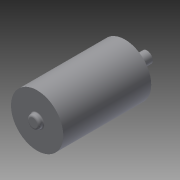
# Autodesk Inventor part: motor
Saved by Autodesk Inventor 2014 SP1 (Build 180222100, 222)
## iProperties
Created: 2014-09-21
Part Number: motor
Material: Générique
Document SubType Name: Modeling
Designer: astralien3000
Density: 1 g/cm^3
Appearance: Par défaut
d0: 25,000 mm
d1: 42,000 mm
d2: 0,00 deg
d3: 7,000 mm
d4: 2,500 mm
d5: 0,00 deg
d6: 5,500 mm
d7: 8,000 mm
d8: 0,00 deg
d9: 1,500 mm
d10: 8,100 mm
d11: 0,00 deg
d12: 3,000 mm
d13: 9,000 mm
d14: 5,500 mm
d15: 0,00 deg
d16: 6,000 mm
d17: 2,000 mm
d18: 0,00 deg
d19: 1,000 mm
d20: 0,500 mm
d21: 0,500 mm
Author: astralien3000
Autodesk Inventor part; units mm, degrees
ref_plane "YZ Plane" through (0, 0, 0) normal (1, 0, 0) x (0, 1, 0)
ref_plane "XZ Plane" through (0, 0, 0) normal (0, 1, 0) x (-1, 0, 0)
ref_plane "XY Plane" through (0, 0, 0) normal (0, 0, 1) x (1, 0, 0)
sketch "Esquisse1" plane through (0, 0, 0) normal (0, 1, 0) x (-1, 0, 0)
  circle A0 centre (0, 0) radius 12.5
  dimension "d0" = 25
  constraints: 1 centre point, 1 coincident
  measures "d0" diameter of A0
extrude "Extrusion1" add sketch "Esquisse1" along normal blind 42
sketch "Esquisse2" plane through (0, 42, 0) normal (0, 1, 0) x (1, 0, 0)
  circle A0 centre (0, 0) radius 12.5 projected
  circle A1 centre (0, 0) radius 3.5
  dimension "d3" = 7
  constraints: 1 centre point, 1 coincident
  measures "d3" diameter of A1
extrude "Extrusion2" add sketch "Esquisse2" along normal blind 2.5 contours A1
sketch "Esquisse3" plane through (0, 44.5, 0) normal (0, 1, 0) x (1, 0, 0)
  circle A0 centre (0, 0) radius 3.5 projected
  circle A1 centre (0, 0) radius 2.75
  dimension "d6" = 5.5
  constraints: 1 centre point, 1 coincident
  measures "d6" diameter of A1
extrude "Extrusion3" add sketch "Esquisse3" along normal blind 8 contours A1
sketch "Esquisse4" plane through (0, 52.5, 0) normal (0, 1, 0) x (1, 0, 0)
  circle A0 centre (0, 0) radius 2.75 projected
  line L0 (-2.3049, 1.5) -> (2.3049, 1.5)
  arc A1 (-2.3049, 1.5) -> (2.3049, 1.5) centre (0, 0) ccw
  arc A2 (2.3049, 1.5) -> (-2.3049, 1.5) centre (0, 0) ccw
  dimension "d9" = 1.5
  constraints: 6 point on circle, 2 centre point, 2 end point, 1 coincident, 1 concentric, 1 horizontal
  measures "d9" distance from line of L0 A0.centre
extrude "Extrusion4" cut sketch "Esquisse4" against normal blind 8.1 contours L0 A0 picked at (0.6217, 1.6736)
sketch "Esquisse5" plane through (0, 42, 0) normal (0, 1, 0) x (1, 0, 0)
  circle A0 centre (0, 0) radius 12.5 projected
  circle A1 centre (-9, 0) radius 1.5
  circle A2 centre (9, 0) radius 1.5
  line L0 (0, 0) -> (0, 12.5) construction
  line L1 (0, 0) -> (-12.5, 0) construction
  dimension "d12" = 3
  dimension "d13" = 9
  constraints: 4 end point, 2 centre point, 2 point on circle, 1 perpendicular, 1 point on line, 1 vertical, 1 other
  measures "d12" diameter of A1
  measures "d13" distance from line of A1.centre L0
extrude "Extrusion5" cut sketch "Esquisse5" against normal blind 5.5 contours A1 | A2
sketch "Esquisse6" plane through (0, 0, 0) normal (0, -1, 0) x (1, 0, 0)
  circle A0 centre (0, 0) radius 12.5 projected
  circle A1 centre (0, 0) radius 3
  dimension "d16" = 6
  constraints: 1 centre point, 1 coincident
  measures "d16" diameter of A1
extrude "Extrusion6" add sketch "Esquisse6" along normal blind 2 contours A1
fillet "Congé1" radius 1 1 edges at (-3, -2, 0)
fillet "Congé2" radius 0.5 1 edges at (-3, 0, 0)
fillet "Congé3" radius 0.5 1 edges at (-3.5, 44.5, 0)
